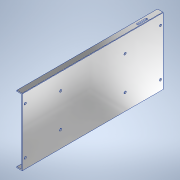
# Autodesk Inventor part: memesat shear panel type 1
Saved by Autodesk Inventor 2022 (Build 260153000, 153)
## iProperties
Created: 2020-02-20
Part Number: memesat shear panel type 1
Material: Aluminum 6061
Document SubType Name: Modeling
Designer: UGA SSRL
Density: 2.7 g/cm^3
Appearance: Aluminum - Flat
Mass: 42.7023 g
Surface Area: 178.409 cm^2
Volume: 15.8157 cm^3
Author: UGA SSRL
Autodesk Inventor part; units mm, degrees
ref_plane "YZ Plane" through (0, 0, 0) normal (1, 0, 0) x (0, 1, 0)
ref_plane "XZ Plane" through (0, 0, 0) normal (0, 1, 0) x (-1, 0, 0)
ref_plane "XY Plane" through (0, 0, 0) normal (0, 0, 1) x (1, 0, 0)
sketch "Sketch1" plane through (0, 0, 0) normal (1, 0, 0) x (0, 1, 0)
  line L0 (48, 50) -> (-48, 50)
  line L1 (-48, 50) -> (-48, -50)
  line L2 (-48, -50) -> (48, -50)
  line L3 (48, -50) -> (48, 50)
  point P0 (0, 0)
  dimension "d0" = 96
  dimension "d1" = 100
  dimension "d2" = 50
  dimension "d3" = 48
  constraints: 8 end point, 2 parallel, 1 horizontal, 1 perpendicular
  measures "d0" distance of L2.end L1.end
  measures "d1" distance of L0.end L1.end
  measures "d2" distance from line of L2 point (0, 0)
  measures "d3" distance from line of L3 point (0, 0)
extrude "Extrusion1" add sketch "Sketch1" along normal blind 1.5
sketch "Sketch2" plane through (0, -48, 50) normal (0, 0, 1) x (1, 0, 0)
  line L0 (0, 96) -> (1.5, 96) projected
  line L1 (1.5, 96) -> (-7, 96)
  line L2 (-7, 96) -> (-7, 0)
  line L3 (-7, 0) -> (1.5, 0)
  line L4 (1.5, 0) -> (1.5, 96)
  point P0 (0, 48)
  dimension "d6" = 8.5
  dimension "d7" = 96
  constraints: 8 end point, 2 perpendicular, 1 horizontal, 1 vertical
  measures "d6" distance of L0.end L1.end
  measures "d7" distance of L1.end L2.end
extrude "Extrusion2" add sketch "Sketch2" against normal blind 1.5
mirror "Mirror1" about plane through (0, 0, 0) normal (0, 0, 1) of "Extrusion2"
fillet "Fillet1" radius 0.5 2 edges at (1.5, 0, 50) (1.5, 0, -50)
sketch "Sketch12" plane through (-7, -48, 48.5) normal (0, -1, 0) x (1, 0, 0)
  arc A0 (8, -98.5) -> (8.5, -98) centre (8, -98) ccw projected
  line L0 (8.5, 1) -> (8.5, -98) projected
  arc A1 (8.5, 1) -> (8, 1.5) centre (8, 1) ccw projected
  line L1 (0, 1.5) -> (8, 1.5) projected
  line L2 (0, 1.5) -> (0, 0) projected
  line L3 (7, 0) -> (0, 0) projected
  line L4 (7, 0) -> (7, -97) projected
  line L5 (7, -97) -> (0, -97) projected
  line L6 (0, -98.5) -> (0, -97) projected
  line L7 (0, -98.5) -> (8, -98.5) projected
  point P0 (7, -48.5)
extrude "Extrusion8" add sketch "Sketch12" along normal blind 56.75
sketch "Sketch13" plane through (-7, 48, 48.5) normal (0, 1, 0) x (1, 0, 0)
  arc A0 (8.5, 98) -> (8, 98.5) centre (8, 98) ccw projected
  line L0 (0, 98.5) -> (8, 98.5) projected
  line L1 (0, 98.5) -> (0, 97) projected
  line L2 (0, 97) -> (7, 97) projected
  line L3 (7, 97) -> (7, 0) projected
  line L4 (0, 0) -> (7, 0) projected
  line L5 (0, -1.5) -> (0, 0) projected
  line L6 (8, -1.5) -> (0, -1.5) projected
  arc A1 (8, -1.5) -> (8.5, -1) centre (8, -1) ccw projected
  line L7 (8.5, 98) -> (8.5, -1) projected
  point P0 (7, 48.5)
extrude "Extrusion9" add sketch "Sketch13" along normal blind 56.75
sketch "Sketch14" plane through (1.5, 0, 0) normal (1, 0, 0) x (0, 0, -1)
  line L0 (49.5, -104.75) -> (49.5, 104.75) projected
  line L1 (-49.5, 104.75) -> (49.5, 104.75) projected
  line L2 (-49.5, 104.75) -> (-49.5, -104.75) projected
  line L3 (49.5, -104.75) -> (-49.5, -104.75) projected
  line L4 (0, 0) -> (-23.5475, 0) construction
  point P0 (35, -100.75)
  point P1 (-35, -100.75)
  point P2 (35, 100.75)
  point P3 (-35, 100.75)
  dimension "d88" = 70
  dimension "d89" = 35
  dimension "d90" = 4
  constraints: 2 end point, 2 symmetric about line, 1 horizontal, 1 horizontal alignment
  measures "d88" distance of point (-35, -100.75) point (35, -100.75)
  measures "d89" horizontal distance of point (-35, -100.75) L4.start
  measures "d90" distance from line of L3 point (35, -100.75)
hole "Hole6" at (1.5, -100.75, -35) at (1.5, -100.75, 35) at (1.5, 100.75, -35) at (1.5, 100.75, 35) direction (-1, 0, 0) diameter 3.454 end through all clearance for "Flat Head Machine Screw (82)" size "#4" standard "Ansi Unified Screw Threads"
sketch "Sketch15" plane through (1.5, 0, 0) normal (1, 0, 0) x (0, 0, -1)
  circle A0 centre (25, -48) radius 1.727 projected
  circle A1 centre (-25, -48) radius 1.727 projected
  circle A2 centre (25, 48) radius 1.727 projected
  circle A3 centre (-25, 48) radius 1.727 projected
  point P0 (0, 0)
hole "Hole7" at (1.5, -48, -25) at (1.5, -48, 25) at (1.5, 48, -25) at (1.5, 48, 25) direction (-1, 0, 0) diameter 3.454 end through all clearance for "Flat Head Machine Screw (82)" size "#4" standard "Ansi Unified Screw Threads"
sketch "Sketch16" plane through (0, 0, 0) normal (-1, 0, 0) x (0, 0, 1)
  line L0 (38.5, 69.75) -> (48.5, 69.75)
  line L1 (48.5, 69.75) -> (48.5, 84.75)
  line L2 (48.5, 84.75) -> (38.5, 84.75)
  line L3 (38.5, 84.75) -> (38.5, 69.75)
  circle A0 centre (-25, 48) radius 1.727 projected
  circle A1 centre (-25, -48) radius 1.727 projected
  circle A2 centre (25, -48) radius 1.727 projected
  circle A3 centre (25, 48) radius 1.727 projected
  circle A4 centre (-35, 100.75) radius 1.727 projected
  circle A5 centre (-35, -100.75) radius 1.727 projected
  circle A6 centre (35, -100.75) radius 1.727 projected
  circle A7 centre (35, 100.75) radius 1.727 projected
  line L4 (-48.5, 104.75) -> (-48.5, -104.75) projected
  line L5 (48.5, -104.75) -> (-48.5, -104.75) projected
  line L6 (48.5, -104.75) -> (48.5, 104.75) projected
  line L7 (-48.5, 104.75) -> (48.5, 104.75) projected
  line L8 (48.5, -104.75) -> (48.5, 104.75) projected
  point P0 (0, 0)
  dimension "d105" = 10
  dimension "d106" = 15
  dimension "d107" = 20
  constraints: 8 end point, 2 parallel, 1 horizontal, 1 perpendicular, 1 point on line
  measures "d105" distance of L0.start L0.end
  measures "d106" distance of L2.end L0.start
  measures "d107" distance between parallel lines of L2 L7
extrude "Extrusion10" add sketch "Sketch16" along normal blind 0.8 contours L3 L2 L1 L0
sketch "Sketch17" plane through (-0.8, 0, 0) normal (-1, 0, 0) x (0, 0, 1)
  line L0 (38.5, 69.75) -> (48.5, 69.75) projected
  line L1 (48.5, 84.75) -> (48.5, 69.75) projected
  line L2 (48.5, 84.75) -> (38.5, 84.75) projected
  line L3 (38.5, 84.75) -> (38.5, 69.75) projected
  line L4 (38.5, 69.75) -> (48.5, 69.75) projected
  point P0 (0, 0)
  point P1 (42.9, 75.25)
  point P2 (42.9, 79.25)
  dimension "d110" = 4
  dimension "d111" = 5.5
  dimension "d123" = 5.6
  constraints: 1 vertical alignment
  measures "d110" distance of point (42.9, 79.25) point (42.9, 75.25)
  measures "d111" distance from line of L0 point (42.9, 75.25)
  measures "d123" distance from line of L1 point (42.9, 75.25)
hole "Hole8" at (-0.8, 75.25, 42.9) at (-0.8, 79.25, 42.9) direction (1, 0, 0) diameter 1.1811 depth 1.651 thread size "0-80 UNF" class "2B" standard "ANSI Unified Screw Threads"
mirror "Mirror2" about plane through (0, 0, 0) normal (0, 0, 1) of "Extrusion10", "Hole8"
sketch "Sketch18" plane through (0, -48, 48.5) normal (0, 0, -1) x (-1, 0, 0)
  line L0 (0.8, 132.75) -> (0.8, 117.75) projected
  line L1 (0, 132.75) -> (0.8, 132.75) projected
  line L2 (0.8, 132.75) -> (3.8, 132.75)
  line L3 (3.8, 132.75) -> (3.8, 117.75)
  line L4 (3.8, 117.75) -> (0.8, 117.75)
  line L5 (0.8, 117.75) -> (0.8, 132.75)
  point P0 (0, 48)
  dimension "d119" = 3
  dimension "d120" = 15
  constraints: 8 end point, 2 parallel, 1 horizontal, 1 perpendicular
  measures "d119" distance of L3.end L4.end
  measures "d120" distance of L2.end L3.end
extrude "Extrusion11" cut sketch "Sketch18" against normal through all
mirror "Mirror3" about plane through (0, 0, 0) normal (0, 0, 1) of "Extrusion11"
chamfer "Chamfer1" distance 2 angle 45 4 edges at (-0.4, 69.75, -38.5) (-0.4, 84.75, -38.5) (-0.4, 69.75, 38.5) (-0.4, 84.75, 38.5)
equation "\"d2\" = 0.5 * d1"
equation "\"d3\" = 0.5 * d0"
equation "\"d89\" = 0.5 * d88"
body "Solid1"
